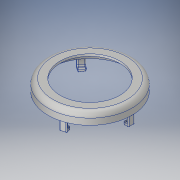
# Autodesk Inventor part: seal cap
Saved by Autodesk Inventor 2018 (Build 220112000, 112)
## iProperties
Created: 2018-02-28
Part Number: seal cap
Material: Aluminum 6061
Document SubType Name: Modeling
Designer: 238438
Density: 2.7 g/cm^3
Appearance: Aluminum - Flat
Author: 238438
Autodesk Inventor part; units mm, degrees
ref_plane "YZ Plane" through (0, 0, 0) normal (1, 0, 0) x (0, 1, 0)
ref_plane "XZ Plane" through (0, 0, 0) normal (0, 1, 0) x (-1, 0, 0)
ref_plane "XY Plane" through (0, 0, 0) normal (0, 0, 1) x (1, 0, 0)
sketch "Sketch1" plane through (0, 0, 0) normal (0, 1, 0) x (-1, 0, 0)
  circle A0 centre (0, 0) radius 6.096
  circle A1 centre (0, 0) radius 8.5725
  dimension "d0" = 12.192
  dimension "d1" = 17.145
  constraints: 2 centre point, 2 coincident
  measures "d0" diameter of A0
  measures "d1" diameter of A1
extrude "Extrusion1" add sketch "Sketch1" along normal blind 2.286
shell "Shell1" thickness 0.4445 removed faces 2 at (-6.0171, 1.524, -0.9779) at (-7.664, 0, -0.6838)
fillet "Fillet1" radius 1.016 1 edges at (8.5725, 2.286, 0)
sketch "Sketch2" plane through (0, 0, 0) normal (0, -1, 0) x (1, 0, 0)
  circle A0 centre (0, 0) radius 8.5725 projected
  line L0 (8.5455, 0.6802) -> (8.128, 0.6802)
  line L1 (8.128, 0.6802) -> (8.128, -0.6284)
  line L2 (8.128, -0.6284) -> (8.5455, -0.6284)
  line L3 (8.5455, -0.6284) -> (8.5455, 0.6802)
  constraints: 8 end point, 2 parallel, 1 horizontal, 1 perpendicular, 2 other
extrude "Extrusion2" add sketch "Sketch2" along normal blind 1.905 contours L3 L2 L1 L0
sketch "Sketch3" plane through (8.128, 0, 0) normal (-1, 0, 0) x (0, 0, 1)
  line L0 (-0.6284, 0) -> (-0.6284, -1.905) projected
  line L1 (0.6802, -1.905) -> (-0.6284, -1.905)
  line L2 (-0.6284, -1.905) -> (-0.6284, -1.1795)
  line L3 (-0.6284, -1.1795) -> (0.6802, -1.1795)
  line L4 (0.6802, -1.1795) -> (0.6802, -1.905)
  point P0 (0, 0)
  constraints: 8 end point, 2 parallel, 1 horizontal, 1 perpendicular, 1 point on line
extrude "Extrusion3" add sketch "Sketch3" along normal blind 0.6477
fillet "Fillet2" radius 0.1905 14 edges at (8.5455, -1.905, 0.0259) (7.4803, -1.905, 0.0259) (7.4803, -1.1795, 0.0259) (8.128, -1.1795, 0.0259) (7.8041, -1.1795, 0.6802) (7.4803, -1.5422, 0.6802) (8.0129, -1.905, 0.6802) (8.5455, -0.9525, 0.6802) (8.128, -0.5897, 0.6802) (7.4803, -1.5422, -0.6284) (7.8041, -1.1795, -0.6284) (8.5455, -0.9525, -0.6284) (8.128, -0.5897, -0.6284) (8.0129, -1.905, -0.6284)
pattern_circular "Circular Pattern1" count 5 over 360 about axis through (0, 0, 0) along (0, 1, 0) of "Fillet2", "Extrusion2", "Extrusion3"
body "Solid1"
